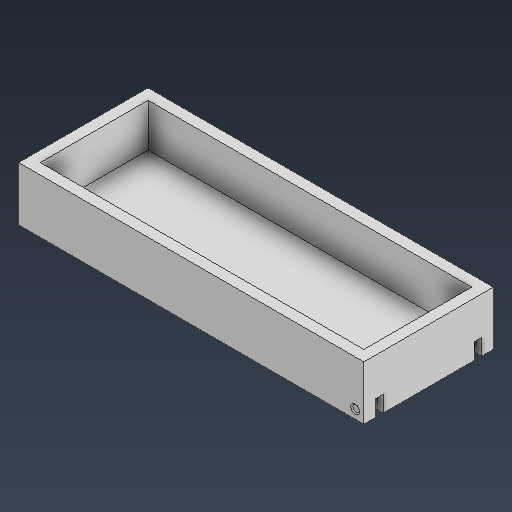
# Autodesk Inventor part: GiveBox
Saved by Autodesk Inventor 2021 (Build 250183000, 183)
## iProperties
Created: 2020-08-04
Part Number: GiveBox
Material: Generic
Document SubType Name: Modeling
Designer: karim
Density: 1 g/cm^3
Appearance: Default
Author: karim
Autodesk Inventor part; units mm, degrees
ref_plane "YZ Plane" through (0, 0, 0) normal (1, 0, 0) x (0, 1, 0)
ref_plane "XZ Plane" through (0, 0, 0) normal (0, 1, 0) x (-1, 0, 0)
sketch "Sketch1" plane through (0, 0, 0) normal (0, 1, 0) x (-1, 0, 0)
  line L0 (150, 50) -> (-150, 50)
  line L1 (-150, 50) -> (-150, -50)
  line L2 (-150, -50) -> (150, -50)
  line L3 (150, -50) -> (150, 50)
  line L4 (150, 50) -> (-150, -50) construction
  line L5 (-150, 50) -> (150, -50) construction
  line L6 (160, 60) -> (-160, 60)
  line L7 (-160, 60) -> (-160, -60)
  line L8 (-160, -60) -> (160, -60)
  line L9 (160, -60) -> (160, 60)
  point P0 (0, 0)
  dimension "d0" = 100
  dimension "d1" = 300
  dimension "d2" = 10
  constraints: 20 end point, 4 parallel, 2 midpoint, 2 perpendicular, 1 horizontal, 3 other
  measures "d0" distance of L0.end L1.end
  measures "d1" distance of L1.end L2.end
  measures "d2" distance between parallel lines of L3 L9
extrude "Extrusion1" add sketch "Sketch1" along normal blind 10 contours L3 L2 L1 L0
extrude "Extrusion2" add sketch "Sketch1" along normal blind 50
sketch "Sketch2" plane through (160, 0, -60) normal (0, 0, -1) x (-1, 0, 0)
  line L0 (0, 0) -> (0, 50) projected
  line L1 (0, 0) -> (0, 3.5)
  line L2 (0, 3.5) -> (3.5, 3.5)
  line L3 (3.5, 3.5) -> (7.9901, 7.9901)
  circle A0 centre (7.9901, 7.9901) radius 3.175
  point P0 (160, 0)
  dimension "d7" = 3.5
  dimension "d8" = 3.5
  dimension "d9" = 6.35
  dimension "d10" = 135
  dimension "d11" = 6.35
  constraints: 6 end point, 1 centre point, 1 coincident, 1 perpendicular, 1 point on line
  measures "d7" distance of L0.start L1.end
  measures "d8" distance of L1.end L2.end
  measures "d9" distance of L2.end L3.end
  measures "d10" angle of L3 L2
  measures "d11" diameter of A0
extrude "Extrusion3" cut sketch "Sketch2" against normal blind 150
fillet "Fillet1" radius 1 2 edges at (155.1849, 7.9901, -60) (155.1849, 7.9901, 60)
sketch "Sketch3" plane through (160, 0, 60) normal (1, 0, 0) x (0, 0, -1)
  line L0 (0, 0) -> (0, 50) projected
  line L1 (0, 0) -> (11, 0)
  line L2 (120, 0) -> (0, 0) projected
  line L3 (11, 0) -> (17.8, 0)
  line L4 (17.8, 0) -> (17.8, 15)
  line L5 (17.8, 15) -> (11, 15)
  line L6 (11, 15) -> (11, 0)
  line L7 (120, 0) -> (120, 50) projected
  line L8 (120, 0) -> (109, 0)
  line L9 (109, 0) -> (102.2, 0)
  line L10 (102.2, 0) -> (102.2, 15)
  line L11 (102.2, 15) -> (109, 15)
  line L12 (109, 15) -> (109, 0)
  point P0 (60, 0)
  point P1 (17.8, 0)
  dimension "d15" = 11
  dimension "d16" = 6.8
  dimension "d17" = 15
  dimension "d18" = 11
  dimension "d19" = 6.8
  constraints: 20 end point, 6 point on line, 5 perpendicular
  measures "d15" distance of L0.start L1.end
  measures "d16" distance of L1.end L3.end
  measures "d17" distance of L3.end L4.end
  measures "d18" distance of L2.start L8.end
  measures "d19" distance of L8.end L9.end
extrude "Extrusion4" cut sketch "Sketch3" against normal blind 13
ref_plane "Work Plane1" through (-150, 50, -42.2) normal (0, 0, 1) x (1, 0, 0)
sketch "Sketch4" plane through (-150, 50, -42.2) normal (0, 0, 1) x (1, 0, 0)
  circle A0 centre (302.0099, -42.0099) radius 4.175 projected
  line L0 (300, -38.3505) -> (300, -37.0005)
  line L1 (300, -39.552) -> (300, 0) projected
  line L2 (297, -50) -> (297, -40) projected
  arc A1 (300, -37.0005) -> (297, -40) centre (299.8581, -39.8585) ccw
  line L3 (297, -40) -> (297.4, -40)
  line L4 (299.552, -40) -> (0, -40) projected
  line L5 (300, -37.0005) -> (300, -37.4005)
  arc A2 (300, -37.4005) -> (297.4, -40) centre (300.0042, -40.0047) ccw
  point P0 (150, -50)
  dimension "d23" = 1.35
  dimension "d24" = 0.4
  dimension "d25" = 0.4
  constraints: 6 end point, 4 point on circle, 3 point on line, 2 centre point, 2 other
  measures "d23" distance of L0.start L0.end
  measures "d24" distance of L2.end L3.end
  measures "d25" distance of L0.end L5.end
extrude "Extrusion5" add sketch "Sketch4" along normal blind 84.4 contours A2 L3 A1 L0
sketch "Sketch5" plane through (0, 10, 0) normal (0, 1, 0) x (1, 0, 0)
  line L0 (147, 49) -> (147, 42.2) projected
  line L1 (147, 49) -> (144, 49)
  line L2 (144, 49) -> (144, 42.2)
  line L3 (144, 42.2) -> (147, 42.2)
  line L4 (147, 42.2) -> (147, 49)
  point P0 (0, 0)
  dimension "d28" = 3
  constraints: 8 end point, 2 parallel, 1 horizontal, 1 perpendicular
  measures "d28" distance of L3.end L2.end
extrude "Extrusion6" cut sketch "Sketch5" against normal blind 84.4
sketch "Sketch6" plane through (0, 10, 0) normal (0, 1, 0) x (1, 0, 0)
  line L0 (147, -49) -> (147, -42.2) projected
  line L1 (147, -49) -> (144, -49)
  line L2 (144, -49) -> (144, -42.2)
  line L3 (144, -42.2) -> (147, -42.2)
  line L4 (147, -42.2) -> (147, -49)
  point P0 (0, 0)
  dimension "d31" = 3
  constraints: 8 end point, 2 parallel, 1 horizontal, 1 perpendicular
  measures "d31" distance of L2.end L3.end
extrude "Extrusion7" cut sketch "Sketch6" against normal blind 84.4
body "Solid1"
